Autodesk Inventor part; units mm, degrees
(part 2 of 2)
sketch "Schizzo14" plane through (0, 0, -0.55) normal (0, 0, -1) x (-1, 0, 0)
  line L0 (-11.7172, -24.6082) -> (11.7172, -24.6082) construction
  line L1 (11.7172, -24.6082) -> (11.7172, -27.25) construction
  line L2 (11.7172, -27.25) -> (-11.7172, -27.25) construction
  line L3 (-11.7172, -27.25) -> (-11.7172, -24.6082) construction
  line L4 (-15, -27.75) -> (15, -27.75) construction
  line L5 (-9.3882, -26.6973) -> (-10.265, -26.6973)
  line L6 (-10.265, -26.6973) -> (-10.265, -26.4931)
  line L7 (-10.265, -26.4931) -> (-9.9392, -26.4931)
  line L8 (-9.9392, -26.4931) -> (-9.9392, -25.1528)
  line L9 (-9.9392, -25.1528) -> (-10.265, -25.1528)
  line L10 (-10.265, -25.1528) -> (-10.265, -24.9696)
  spline S0 degree 2 poles (-10.265, -24.9696) (-10.0802, -24.9696) (-9.9052, -24.8529) (-9.8938, -24.6908) knots 0 0 0 1 2 2 2
  line L11 (-9.8938, -24.6908) -> (-9.7075, -24.6908)
  line L12 (-9.7075, -24.6908) -> (-9.7075, -26.4931)
  line L13 (-9.7075, -26.4931) -> (-9.3882, -26.4931)
  line L14 (-9.3882, -26.4931) -> (-9.3882, -26.6973)
  line L15 (-8.6702, -26.6973) -> (-8.9587, -26.6973)
  line L16 (-8.9587, -26.6973) -> (-8.9587, -26.3148)
  line L17 (-8.9587, -26.3148) -> (-8.6702, -26.3148)
  line L18 (-8.6702, -26.3148) -> (-8.6702, -26.6973)
  line L19 (-7.1791, -24.9972) -> (-7.9554, -26.6973)
  line L20 (-7.9554, -26.6973) -> (-8.2131, -26.6973)
  line L21 (-8.2131, -26.6973) -> (-7.3914, -24.9323)
  line L22 (-7.3914, -24.9323) -> (-8.3201, -24.9323)
  line L23 (-8.3201, -24.9323) -> (-8.3201, -24.6973)
  line L24 (-8.3201, -24.6973) -> (-7.1791, -24.6973)
  line L25 (-7.1791, -24.6973) -> (-7.1791, -24.9972)
  line L26 (-5.829, -24.9972) -> (-6.6053, -26.6973)
  line L27 (-6.6053, -26.6973) -> (-6.863, -26.6973)
  line L28 (-6.863, -26.6973) -> (-6.0413, -24.9323)
  line L29 (-6.0413, -24.9323) -> (-6.97, -24.9323)
  line L30 (-6.97, -24.9323) -> (-6.97, -24.6973)
  line L31 (-6.97, -24.6973) -> (-5.829, -24.6973)
  line L32 (-5.829, -24.6973) -> (-5.829, -24.9972)
  line L33 (-5.3395, -24.6082) -> (-5.3914, -25.3861)
  line L34 (-5.3914, -25.3861) -> (-5.5502, -25.3861)
  line L35 (-5.5502, -25.3861) -> (-5.6021, -24.6082)
  line L36 (-5.6021, -24.6082) -> (-5.3395, -24.6082)
  line L37 (-4.8857, -24.6082) -> (-4.9376, -25.3861)
  line L38 (-4.9376, -25.3861) -> (-5.0964, -25.3861)
  line L39 (-5.0964, -25.3861) -> (-5.1483, -24.6082)
  line L40 (-5.1483, -24.6082) -> (-4.8857, -24.6082)
  line L41 (-2.8225, -26.6973) -> (-3.6994, -26.6973)
  line L42 (-3.6994, -26.6973) -> (-3.6994, -26.4931)
  line L43 (-3.6994, -26.4931) -> (-3.3736, -26.4931)
  line L44 (-3.3736, -26.4931) -> (-3.3736, -25.1528)
  line L45 (-3.3736, -25.1528) -> (-3.6994, -25.1528)
  line L46 (-3.6994, -25.1528) -> (-3.6994, -24.9696)
  spline S1 degree 2 poles (-3.6994, -24.9696) (-3.5146, -24.9696) (-3.3395, -24.8529) (-3.3282, -24.6908) knots 0 0 0 1 2 2 2
  line L47 (-3.3282, -24.6908) -> (-3.1418, -24.6908)
  line L48 (-3.1418, -24.6908) -> (-3.1418, -26.4931)
  line L49 (-3.1418, -26.4931) -> (-2.8225, -26.4931)
  line L50 (-2.8225, -26.4931) -> (-2.8225, -26.6973)
  spline S2 degree 2 poles (-1.3541, -26.049) (-1.3541, -26.203) (-1.4465, -26.4639) (-1.5227, -26.5515) knots 0 0 0 1 2 2 2
  spline S3 degree 2 poles (-1.5227, -26.5515) (-1.6037, -26.6438) (-1.8047, -26.7395) (-1.9263, -26.7395) knots 0 0 0 1 2 2 2
  spline S4 degree 2 poles (-1.9263, -26.7395) (-2.0478, -26.7395) (-2.2472, -26.6487) (-2.3233, -26.5579) knots 0 0 0 1 2 2 2
  spline S5 degree 2 poles (-2.3233, -26.5579) (-2.4157, -26.4494) (-2.5211, -26.0847) (-2.5211, -25.8189) knots 0 0 0 1 2 2 2
  spline S6 degree 2 poles (-2.5211, -25.8189) (-2.5211, -25.5579) (-2.4238, -25.1382) (-2.3233, -24.9826) knots 0 0 0 1 2 2 2
  spline S7 degree 2 poles (-2.3233, -24.9826) (-2.2261, -24.8302) (-1.9165, -24.66) (-1.7139, -24.66) knots 0 0 0 1 2 2 2
  spline S8 degree 2 poles (-1.7139, -24.66) (-1.654, -24.66) (-1.5502, -24.673) (-1.5097, -24.6876) knots 0 0 0 1 2 2 2
  line L51 (-1.5097, -24.6876) -> (-1.5097, -24.9453)
  line L52 (-1.5097, -24.9453) -> (-1.5211, -24.9453)
  spline S9 degree 2 poles (-1.5211, -24.9453) (-1.5535, -24.9259) (-1.6767, -24.8918) (-1.7464, -24.8918) knots 0 0 0 1 2 2 2
  spline S10 degree 2 poles (-1.7464, -24.8918) (-1.9716, -24.8918) (-2.2472, -25.2289) (-2.2731, -25.5596) knots 0 0 0 1 2 2 2
  spline S11 degree 2 poles (-2.2731, -25.5596) (-2.1872, -25.4931) (-2.0057, -25.4202) (-1.8987, -25.4202) knots 0 0 0 1 2 2 2
  spline S12 degree 2 poles (-1.8987, -25.4202) (-1.7934, -25.4202) (-1.6361, -25.4672) (-1.5502, -25.5385) knots 0 0 0 1 2 2 2
  spline S13 degree 2 poles (-1.5502, -25.5385) (-1.4514, -25.6212) (-1.3541, -25.8772) (-1.3541, -26.049) knots 0 0 0 1 2 2 2
  spline S14 degree 2 poles (-1.5989, -26.0604) (-1.5989, -25.9372) (-1.6572, -25.7703) (-1.722, -25.7119) knots 0 0 0 1 2 2 2
  spline S15 degree 2 poles (-1.722, -25.7119) (-1.769, -25.6698) (-1.889, -25.6422) (-1.9522, -25.6422) knots 0 0 0 1 2 2 2
  spline S16 degree 2 poles (-1.9522, -25.6422) (-2.0365, -25.6422) (-2.1953, -25.6989) (-2.2731, -25.7524) knots 0 0 0 1 2 2 2
  spline S17 degree 2 poles (-2.2731, -25.7524) (-2.2763, -25.7816) (-2.278, -25.8367) (-2.278, -25.8788) knots 0 0 0 1 2 2 2
  spline S18 degree 2 poles (-2.278, -25.8788) (-2.278, -26.0863) (-2.205, -26.3408) (-2.1499, -26.4072) knots 0 0 0 1 2 2 2
  spline S19 degree 2 poles (-2.1499, -26.4072) (-2.0981, -26.4704) (-1.9878, -26.5207) (-1.9246, -26.5207) knots 0 0 0 1 2 2 2
  spline S20 degree 2 poles (-1.9246, -26.5207) (-1.7788, -26.5207) (-1.5989, -26.2905) (-1.5989, -26.0604) knots 0 0 0 1 2 2 2
  line L53 (-0.4157, -27.25) -> (-0.6929, -27.25)
  spline S21 degree 2 poles (-0.6929, -27.25) (-0.9036, -26.9729) (-1.1434, -26.3521) (-1.1434, -25.9291) knots 0 0 0 1 2 2 2
  spline S22 degree 2 poles (-1.1434, -25.9291) (-1.1434, -25.5158) (-0.9052, -24.8853) (-0.6929, -24.6082) knots 0 0 0 1 2 2 2
  line L54 (-0.6929, -24.6082) -> (-0.4157, -24.6082)
  line L55 (-0.4157, -24.6082) -> (-0.4157, -24.6212)
  spline S23 degree 2 poles (-0.4157, -24.6212) (-0.513, -24.72) (-0.6912, -24.9761) (-0.7674, -25.1463) knots 0 0 0 1 2 2 2
  spline S24 degree 2 poles (-0.7674, -25.1463) (-0.8404, -25.3116) (-0.9311, -25.7087) (-0.9311, -25.9291) knots 0 0 0 1 2 2 2
  spline S25 degree 2 poles (-0.9311, -25.9291) (-0.9311, -26.1592) (-0.842, -26.5401) (-0.7674, -26.7119) knots 0 0 0 1 2 2 2
  spline S26 degree 2 poles (-0.7674, -26.7119) (-0.6945, -26.8772) (-0.5081, -27.1447) (-0.4157, -27.237) knots 0 0 0 1 2 2 2
  line L56 (-0.4157, -27.237) -> (-0.4157, -27.25)
  line L57 (1.2488, -26.6973) -> (0.9392, -26.6973)
  line L58 (0.9392, -26.6973) -> (0.3687, -25.9015)
  line L59 (0.3687, -25.9015) -> (0.0964, -25.9015)
  line L60 (0.0964, -25.9015) -> (0.0964, -26.6973)
  line L61 (0.0964, -26.6973) -> (-0.1434, -26.6973)
  line L62 (-0.1434, -26.6973) -> (-0.1434, -24.6973)
  line L63 (-0.1434, -24.6973) -> (0.3201, -24.6973)
  spline S27 degree 2 poles (0.3201, -24.6973) (0.4741, -24.6973) (0.6831, -24.7346) (0.7771, -24.8027) knots 0 0 0 1 2 2 2
  spline S28 degree 2 poles (0.7771, -24.8027) (0.8712, -24.8707) (0.9814, -25.0831) (0.9814, -25.2403) knots 0 0 0 1 2 2 2
  spline S29 degree 2 poles (0.9814, -25.2403) (0.9814, -25.4591) (0.782, -25.7557) (0.6086, -25.827) knots 0 0 0 1 2 2 2
  line L64 (0.6086, -25.827) -> (1.2488, -26.6973)
  spline S30 degree 2 poles (0.7334, -25.2613) (0.7334, -25.1738) (0.6783, -25.0393) (0.6199, -24.9955) knots 0 0 0 1 2 2 2
  spline S31 degree 2 poles (0.6199, -24.9955) (0.5697, -24.9583) (0.4335, -24.9275) (0.3331, -24.9275) knots 0 0 0 1 2 2 2
  line L65 (0.3331, -24.9275) -> (0.0964, -24.9275)
  line L66 (0.0964, -24.9275) -> (0.0964, -25.6795)
  line L67 (0.0964, -25.6795) -> (0.3071, -25.6795)
  spline S32 degree 2 poles (0.3071, -25.6795) (0.4092, -25.6795) (0.5746, -25.639) (0.6313, -25.5758) knots 0 0 0 1 2 2 2
  spline S33 degree 2 poles (0.6313, -25.5758) (0.6831, -25.5207) (0.7334, -25.3651) (0.7334, -25.2613) knots 0 0 0 1 2 2 2
  spline S34 degree 2 poles (2.1434, -26.7362) (1.9522, -26.7362) (1.6361, -26.6066) (1.5227, -26.4753) knots 0 0 0 1 2 2 2
  spline S35 degree 2 poles (1.5227, -26.4753) (1.4092, -26.3424) (1.2877, -25.9502) (1.2877, -25.6957) knots 0 0 0 1 2 2 2
  spline S36 degree 2 poles (1.2877, -25.6957) (1.2877, -25.4542) (1.4092, -25.0717) (1.5227, -24.9356) knots 0 0 0 1 2 2 2
  spline S37 degree 2 poles (1.5227, -24.9356) (1.6329, -24.8043) (1.9554, -24.6617) (2.1467, -24.6617) knots 0 0 0 1 2 2 2
  spline S38 degree 2 poles (2.1467, -24.6617) (2.2374, -24.6617) (2.4044, -24.6908) (2.4806, -24.7168) knots 0 0 0 1 2 2 2
  spline S39 degree 2 poles (2.4806, -24.7168) (2.5405, -24.7362) (2.6896, -24.8075) (2.735, -24.8335) knots 0 0 0 1 2 2 2
  line L68 (2.735, -24.8335) -> (2.735, -25.1544)
  line L69 (2.735, -25.1544) -> (2.7139, -25.1544)
  spline S40 degree 2 poles (2.7139, -25.1544) (2.6702, -25.1106) (2.5746, -25.0312) (2.487, -24.9858) knots 0 0 0 1 2 2 2
  spline S41 degree 2 poles (2.487, -24.9858) (2.4141, -24.9453) (2.2261, -24.8918) (2.1159, -24.8918) knots 0 0 0 1 2 2 2
  spline S42 degree 2 poles (2.1159, -24.8918) (1.8566, -24.8918) (1.5357, -25.3262) (1.5357, -25.6876) knots 0 0 0 1 2 2 2
  spline S43 degree 2 poles (1.5357, -25.6876) (1.5357, -25.8886) (1.6199, -26.19) (1.701, -26.2938) knots 0 0 0 1 2 2 2
  spline S44 degree 2 poles (1.701, -26.2938) (1.7771, -26.3975) (1.9959, -26.5061) (2.1337, -26.5061) knots 0 0 0 1 2 2 2
  spline S45 degree 2 poles (2.1337, -26.5061) (2.2358, -26.5061) (2.4352, -26.4737) (2.5049, -26.4412) knots 0 0 0 1 2 2 2
  line L70 (2.5049, -26.4412) -> (2.5049, -25.9242)
  line L71 (2.5049, -25.9242) -> (2.0883, -25.9242)
  line L72 (2.0883, -25.9242) -> (2.0883, -25.6908)
  line L73 (2.0883, -25.6908) -> (2.7415, -25.6908)
  line L74 (2.7415, -25.6908) -> (2.7415, -26.5644)
  spline S46 degree 2 poles (2.7415, -26.5644) (2.6961, -26.5871) (2.5421, -26.6568) (2.4757, -26.6779) knots 0 0 0 1 2 2 2
  spline S47 degree 2 poles (2.4757, -26.6779) (2.3882, -26.7071) (2.2455, -26.7362) (2.1434, -26.7362) knots 0 0 0 1 2 2 2
  spline S48 degree 2 poles (4.2617, -26.0831) (4.2617, -26.2322) (4.1596, -26.4607) (4.0754, -26.5353) knots 0 0 0 1 2 2 2
  spline S49 degree 2 poles (4.0754, -26.5353) (3.9733, -26.6228) (3.7415, -26.6973) (3.5583, -26.6973) knots 0 0 0 1 2 2 2
  line L75 (3.5583, -26.6973) -> (3.0429, -26.6973)
  line L76 (3.0429, -26.6973) -> (3.0429, -24.6973)
  line L77 (3.0429, -24.6973) -> (3.5194, -24.6973)
  spline S50 degree 2 poles (3.5194, -24.6973) (3.7123, -24.6973) (3.9036, -24.7249) (3.9911, -24.7784) knots 0 0 0 1 2 2 2
  spline S51 degree 2 poles (3.9911, -24.7784) (4.0883, -24.8351) (4.1775, -25.0215) (4.1775, -25.1479) knots 0 0 0 1 2 2 2
  spline S52 degree 2 poles (4.1775, -25.1479) (4.1775, -25.2889) (4.0429, -25.5126) (3.9263, -25.5758) knots 0 0 0 1 2 2 2
  line L78 (3.9263, -25.5758) -> (3.9263, -25.5855)
  spline S53 degree 2 poles (3.9263, -25.5855) (4.0851, -25.6341) (4.2617, -25.8918) (4.2617, -26.0831) knots 0 0 0 1 2 2 2
  spline S54 degree 2 poles (4.0138, -26.0944) (4.0138, -25.981) (3.9554, -25.8351) (3.8679, -25.7832) knots 0 0 0 1 2 2 2
  spline S55 degree 2 poles (3.8679, -25.7832) (3.8112, -25.7508) (3.6767, -25.7314) (3.5535, -25.7314) knots 0 0 0 1 2 2 2
  line L79 (3.5535, -25.7314) -> (3.2828, -25.7314)
  line L80 (3.2828, -25.7314) -> (3.2828, -26.4704)
  line L81 (3.2828, -26.4704) -> (3.4773, -26.4704)
  spline S56 degree 2 poles (3.4773, -26.4704) (3.6345, -26.4704) (3.8144, -26.438) (3.8841, -26.3861) knots 0 0 0 1 2 2 2
  spline S57 degree 2 poles (3.8841, -26.3861) (3.9506, -26.3327) (4.0138, -26.1998) (4.0138, -26.0944) knots 0 0 0 1 2 2 2
  spline S58 degree 2 poles (3.9295, -25.1852) (3.9295, -25.1139) (3.8857, -25.0069) (3.8371, -24.9761) knots 0 0 0 1 2 2 2
  spline S59 degree 2 poles (3.8371, -24.9761) (3.7804, -24.9404) (3.6378, -24.9242) (3.5113, -24.9242) knots 0 0 0 1 2 2 2
  line L82 (3.5113, -24.9242) -> (3.2828, -24.9242)
  line L83 (3.2828, -24.9242) -> (3.2828, -25.5093)
  line L84 (3.2828, -25.5093) -> (3.5535, -25.5093)
  spline S60 degree 2 poles (3.5535, -25.5093) (3.6669, -25.5093) (3.7723, -25.4834) (3.829, -25.4429) knots 0 0 0 1 2 2 2
  spline S61 degree 2 poles (3.829, -25.4429) (3.8841, -25.404) (3.9295, -25.2792) (3.9295, -25.1852) knots 0 0 0 1 2 2 2
  spline S62 degree 2 poles (5.1337, -25.9291) (5.1337, -26.344) (4.8938, -26.9729) (4.6831, -27.25) knots 0 0 0 1 2 2 2
  line L85 (4.6831, -27.25) -> (4.406, -27.25)
  line L86 (4.406, -27.25) -> (4.406, -27.237)
  spline S63 degree 2 poles (4.406, -27.237) (4.4984, -27.1447) (4.688, -26.874) (4.7577, -26.7119) knots 0 0 0 1 2 2 2
  spline S64 degree 2 poles (4.7577, -26.7119) (4.8339, -26.5385) (4.9214, -26.1528) (4.9214, -25.9291) knots 0 0 0 1 2 2 2
  spline S65 degree 2 poles (4.9214, -25.9291) (4.9214, -25.7071) (4.8323, -25.3132) (4.7577, -25.1463) knots 0 0 0 1 2 2 2
  spline S66 degree 2 poles (4.7577, -25.1463) (4.6848, -24.9793) (4.4984, -24.7135) (4.406, -24.6212) knots 0 0 0 1 2 2 2
  line L87 (4.406, -24.6212) -> (4.406, -24.6082)
  line L88 (4.406, -24.6082) -> (4.6831, -24.6082)
  spline S67 degree 2 poles (4.6831, -24.6082) (4.8938, -24.8853) (5.1337, -25.5109) (5.1337, -25.9291) knots 0 0 0 1 2 2 2
  line L89 (6.4773, -26.6973) -> (6.1985, -26.6973)
  line L90 (6.1985, -26.6973) -> (5.8695, -26.1301)
  line L91 (5.8695, -26.1301) -> (5.5324, -26.6973)
  line L92 (5.5324, -26.6973) -> (5.2747, -26.6973)
  line L93 (5.2747, -26.6973) -> (5.7431, -25.9534)
  line L94 (5.7431, -25.9534) -> (5.2796, -25.1965)
  line L95 (5.2796, -25.1965) -> (5.5583, -25.1965)
  line L96 (5.5583, -25.1965) -> (5.8857, -25.7589)
  line L97 (5.8857, -25.7589) -> (6.2196, -25.1965)
  line L98 (6.2196, -25.1965) -> (6.4773, -25.1965)
  line L99 (6.4773, -25.1965) -> (6.0122, -25.9356)
  line L100 (6.0122, -25.9356) -> (6.4773, -26.6973)
  line L101 (7.6394, -26.6973) -> (6.7626, -26.6973)
  line L102 (6.7626, -26.6973) -> (6.7626, -26.4931)
  line L103 (6.7626, -26.4931) -> (7.0883, -26.4931)
  line L104 (7.0883, -26.4931) -> (7.0883, -25.1528)
  line L105 (7.0883, -25.1528) -> (6.7626, -25.1528)
  line L106 (6.7626, -25.1528) -> (6.7626, -24.9696)
  spline S68 degree 2 poles (6.7626, -24.9696) (6.9473, -24.9696) (7.1224, -24.8529) (7.1337, -24.6908) knots 0 0 0 1 2 2 2
  line L107 (7.1337, -24.6908) -> (7.3201, -24.6908)
  line L108 (7.3201, -24.6908) -> (7.3201, -26.4931)
  line L109 (7.3201, -26.4931) -> (7.6394, -26.4931)
  line L110 (7.6394, -26.4931) -> (7.6394, -26.6973)
  line L111 (9.0802, -26.6973) -> (7.97, -26.6973)
  line L112 (7.97, -26.6973) -> (7.97, -26.4137)
  spline S69 degree 2 poles (7.97, -26.4137) (8.09, -26.2889) (8.3039, -26.0571) (8.4044, -25.9323) knots 0 0 0 1 2 2 2
  spline S70 degree 2 poles (8.4044, -25.9323) (8.6102, -25.6811) (8.7609, -25.3797) (8.7609, -25.2192) knots 0 0 0 1 2 2 2
  spline S71 degree 2 poles (8.7609, -25.2192) (8.7609, -25.1349) (8.7139, -25.0085) (8.6718, -24.968) knots 0 0 0 1 2 2 2
  spline S72 degree 2 poles (8.6718, -24.968) (8.6297, -24.9275) (8.5178, -24.887) (8.4514, -24.887) knots 0 0 0 1 2 2 2
  spline S73 degree 2 poles (8.4514, -24.887) (8.3882, -24.887) (8.2553, -24.9226) (8.1953, -24.9502) knots 0 0 0 1 2 2 2
  spline S74 degree 2 poles (8.1953, -24.9502) (8.1434, -24.9729) (8.0494, -25.0377) (8.0203, -25.0604) knots 0 0 0 1 2 2 2
  line L113 (8.0203, -25.0604) -> (8.0073, -25.0604)
  line L114 (8.0073, -25.0604) -> (8.0073, -24.7751)
  spline S75 degree 2 poles (8.0073, -24.7751) (8.0818, -24.7346) (8.3493, -24.6552) (8.4692, -24.6552) knots 0 0 0 1 2 2 2
  spline S76 degree 2 poles (8.4692, -24.6552) (8.7204, -24.6552) (9.0057, -24.9518) (9.0057, -25.2046) knots 0 0 0 1 2 2 2
  spline S77 degree 2 poles (9.0057, -25.2046) (9.0057, -25.3229) (8.9554, -25.5207) (8.9133, -25.6049) knots 0 0 0 1 2 2 2
  spline S78 degree 2 poles (8.9133, -25.6049) (8.8679, -25.6925) (8.7415, -25.8643) (8.6718, -25.9469) knots 0 0 0 1 2 2 2
  spline S79 degree 2 poles (8.6718, -25.9469) (8.5583, -26.0847) (8.2796, -26.3797) (8.1953, -26.4656) knots 0 0 0 1 2 2 2
  line L115 (8.1953, -26.4656) -> (9.0802, -26.4656)
  line L116 (9.0802, -26.4656) -> (9.0802, -26.6973)
  spline S80 degree 2 poles (9.8647, -26.7427) (9.7301, -26.7427) (9.5097, -26.6536) (9.4319, -26.5709) knots 0 0 0 1 2 2 2
  spline S81 degree 2 poles (9.4319, -26.5709) (9.3558, -26.4899) (9.278, -26.2694) (9.278, -26.1447) knots 0 0 0 1 2 2 2
  spline S82 degree 2 poles (9.278, -26.1447) (9.278, -25.9826) (9.4335, -25.7103) (9.5827, -25.6293) knots 0 0 0 1 2 2 2
  line L117 (9.5827, -25.6293) -> (9.5827, -25.6212)
  spline S83 degree 2 poles (9.5827, -25.6212) (9.4498, -25.5353) (9.3217, -25.331) (9.3217, -25.1787) knots 0 0 0 1 2 2 2
  spline S84 degree 2 poles (9.3217, -25.1787) (9.3217, -24.9534) (9.628, -24.6519) (9.863, -24.6519) knots 0 0 0 1 2 2 2
  spline S85 degree 2 poles (9.863, -24.6519) (10.1094, -24.6519) (10.4044, -24.9372) (10.4044, -25.1609) knots 0 0 0 1 2 2 2
  spline S86 degree 2 poles (10.4044, -25.1609) (10.4044, -25.2954) (10.2634, -25.5579) (10.1305, -25.6325) knots 0 0 0 1 2 2 2
  line L118 (10.1305, -25.6325) -> (10.1305, -25.6406)
  spline S87 degree 2 poles (10.1305, -25.6406) (10.2877, -25.7216) (10.4498, -25.955) (10.4498, -26.1398) knots 0 0 0 1 2 2 2
  spline S88 degree 2 poles (10.4498, -26.1398) (10.4498, -26.3959) (10.1159, -26.7427) (9.8647, -26.7427) knots 0 0 0 1 2 2 2
  spline S89 degree 2 poles (10.2018, -26.1657) (10.2018, -26.0425) (10.1143, -25.8967) (9.9911, -25.8221) knots 0 0 0 1 2 2 2
  spline S90 degree 2 poles (9.9911, -25.8221) (9.9489, -25.7962) (9.8128, -25.7362) (9.7269, -25.6973) knots 0 0 0 1 2 2 2
  spline S91 degree 2 poles (9.7269, -25.6973) (9.628, -25.7703) (9.5211, -25.9874) (9.5211, -26.1252) knots 0 0 0 1 2 2 2
  spline S92 degree 2 poles (9.5211, -26.1252) (9.5211, -26.3067) (9.7172, -26.5434) (9.8663, -26.5434) knots 0 0 0 1 2 2 2
  spline S93 degree 2 poles (9.8663, -26.5434) (10.0186, -26.5434) (10.2018, -26.3408) (10.2018, -26.1657) knots 0 0 0 1 2 2 2
  spline S94 degree 2 poles (10.1677, -25.1641) (10.1677, -25.0296) (10.0057, -24.8497) (9.863, -24.8497) knots 0 0 0 1 2 2 2
  spline S95 degree 2 poles (9.863, -24.8497) (9.7301, -24.8497) (9.5632, -25.0101) (9.5632, -25.1479) knots 0 0 0 1 2 2 2
  spline S96 degree 2 poles (9.5632, -25.1479) (9.5632, -25.2468) (9.6491, -25.3845) (9.735, -25.4396) knots 0 0 0 1 2 2 2
  spline S97 degree 2 poles (9.735, -25.4396) (9.7723, -25.4623) (9.9263, -25.5417) (9.9878, -25.5644) knots 0 0 0 1 2 2 2
  spline S98 degree 2 poles (9.9878, -25.5644) (10.0932, -25.4753) (10.1677, -25.2857) (10.1677, -25.1641) knots 0 0 0 1 2 2 2
  point P0 (0, 0)
  point P1 (0, -27.25)
  point P2 (0, -27.75)
  point P3 (0, -27.75)
  dimension "d0" = 34
  dimension "d1" = 55.5
  dimension "d140" = 0.5
  constraints: 3 midpoint, 1 vertical alignment, 2 other
  measures "d140" distance between parallel lines of L4 L2
emboss "Sbalzo2" sketch "Schizzo14" operation add depth 0.05 direction (0, 0, 1)
sketch "Náčrt15" plane through (17, -25.75, 0.55) normal (1, 0, 0) x (0, 0, -1)
  line L0 (1.1, 48.3) -> (4.2, 48.3) projected
  line L1 (3.7728, 48.3) -> (3.7728, 53.5)
  line L2 (3.7728, 53.5) -> (0, 53.5)
  line L3 (0, 53.5) -> (0, -2)
  line L4 (0, -2) -> (3.7728, -2)
  line L5 (3.7728, -2) -> (3.7728, 48.3)
  line L6 (1.1, 4.6) -> (4.2, 4.6) projected
  point P0 (0.55, 25.75)
  point P1 (0, 25.75)
  point P2 (0, -2)
  dimension "d143" = 3.7728
  dimension "d144" = 55.5
  constraints: 10 end point, 4 perpendicular, 2 point on line, 1 coincident, 1 horizontal alignment, 1 midpoint, 1 vertical
  measures "d143" distance of L3.end L4.end
  measures "d144" distance of L2.end L3.end
extrude "Vysunutí11" add sketch "Náčrt15" against normal blind 34 bodies 1
sketch "Náčrt16" plane through (-17, -21.15, -0.55) normal (-1, 0, 0) x (0, 0, 1)
  point P0 (0.55, 21.15)
sketch "Náčrt17" plane through (-17, -25.75, 0.55) normal (-1, 0, 0) x (0, 0, 1)
  line L0 (0, 53.5) -> (-3.7728, 53.5) projected
  line L1 (-3.7728, -2) -> (0, -2) projected
  line L2 (-0.3864, -2) -> (-3.3864, -2)
  line L3 (-3.3864, -2) -> (-3.3864, 2)
  line L4 (-3.3864, 2) -> (-0.3864, 2)
  line L5 (-0.3864, 2) -> (-0.3864, -2)
  line L6 (-0.3864, -2) -> (-3.3864, 2) construction
  line L7 (-3.3864, -2) -> (-0.3864, 2) construction
  line L8 (-3.3864, 49.5) -> (-0.3864, 49.5)
  line L9 (-0.3864, 49.5) -> (-0.3864, 53.5)
  line L10 (-0.3864, 53.5) -> (-3.3864, 53.5)
  line L11 (-3.3864, 53.5) -> (-3.3864, 49.5)
  line L12 (-3.3864, 49.5) -> (-0.3864, 53.5) construction
  line L13 (-0.3864, 49.5) -> (-3.3864, 53.5) construction
  point P0 (-0.55, 25.75)
  point P1 (-1.8864, 53.5)
  point P2 (-1.8864, 53.5)
  point P3 (-1.8864, 0)
  point P4 (-1.8864, -2)
  point P5 (-1.8864, -2)
  point P6 (0, 0)
  point P7 (-1.8864, 51.5)
  point P8 (0, 51.5)
  point P9 (-0.3864, 53.5)
  point P10 (-3.3864, 53.5)
  point P11 (-3.3864, -2)
  point P12 (-0.3864, -2)
  dimension "d151" = 3
  dimension "d152" = 4
  dimension "d153" = 2
  dimension "d154" = 3
  dimension "d155" = 4
  constraints: 24 end point, 8 midpoint, 4 parallel, 2 horizontal, 2 horizontal alignment, 2 perpendicular, 2 vertical alignment
  measures "d151" distance of L3.end L4.end
  measures "d152" distance of L2.end L3.end
  measures "d153" distance of point (-1.886, -2) point (-1.886, 0)
  measures "d154" distance of L10.end L9.end
  measures "d155" distance of L9.end L8.end
extrude "Vysunutí12" add sketch "Náčrt17" along normal blind 20 bodies 1
equation "\"d30\" = d22"
equation "\"d46\" = d33"
equation "\"d71\" = d70"
equation "\"d72\" = d70"
equation "\"d73\" = d70"
equation "\"d75\" = d70"
equation "\"d76\" = d70"
equation "\"d77\" = d70"
equation "\"d78\" = d70"
equation "\"d116\" = d114"
equation "\"d125\" = d124"
equation "\"d126\" = d124"
equation "\"d127\" = d124"
